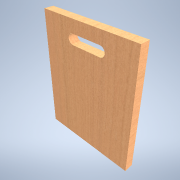
# Autodesk Inventor part: Creat Side
Saved by Autodesk Inventor 2021 (Build 250183000, 183)
## iProperties
Created: 2020-08-15
Part Number: Creat Side
Material: Wood (Cherry)
Document SubType Name: Modeling
Designer: Oghenemarho
Density: 0.63 g/cm^3
Appearance: Cherry - Natural Low Gloss
Author: Oghenemarho
Autodesk Inventor part; units mm, degrees
ref_plane "YZ Plane" through (0, 0, 0) normal (1, 0, 0) x (0, 1, 0)
ref_plane "XZ Plane" through (0, 0, 0) normal (0, 1, 0) x (-1, 0, 0)
ref_plane "XY Plane" through (0, 0, 0) normal (0, 0, 1) x (1, 0, 0)
sketch "Sketch1" plane through (0, 0, 0) normal (0, 0, 1) x (1, 0, 0)
  line L0 (-100, -125) -> (100, -125)
  line L1 (100, -125) -> (100, 125)
  line L2 (100, 125) -> (-100, 125)
  line L3 (-100, 125) -> (-100, -125)
  line L4 (-100, -125) -> (100, 125) construction
  line L5 (100, -125) -> (-100, 125) construction
  point P0 (0, 0)
  dimension "Height" = 250
  dimension "Width" = 200
  constraints: 12 end point, 2 midpoint, 2 parallel, 1 horizontal, 1 perpendicular
  measures "Height" distance of L0.end L1.end
  measures "Width" distance of L0.start L0.end
extrude "Extrusion1" add sketch "Sketch1" along normal blind 19.05
sketch "Sketch2" plane through (0, 0, 19.05) normal (0, 0, 1) x (1, 0, 0)
  line L0 (-30, 90) -> (30, 90) construction
  line L1 (-30, 80) -> (30, 80)
  line L2 (30, 100) -> (-30, 100)
  arc A0 (-30, 100) -> (-30, 80) centre (-30, 90) ccw
  arc A1 (30, 80) -> (30, 100) centre (30, 90) ccw
  line L3 (100, 125) -> (-100, 125) projected
  point P0 (0, 0)
  point P1 (0, 90)
  dimension "d4" = 30
  dimension "d5" = 20
  dimension "d6" = 25
  constraints: 8 end point, 4 point on circle, 4 tangent, 2 centre point, 1 horizontal, 1 midpoint, 1 parallel, 1 vertical alignment
  measures "d4" distance of point (0, 90) L0.end
  measures "d5" diameter of A1
  measures "d6" distance between parallel lines of L3 L2
extrude "Extrusion2" cut sketch "Sketch2" against normal up to surface (19.05 mm away)
equation "\"d7\" = thickness"
equation "\"thickness\" = 19.05"
body "Solid1"
